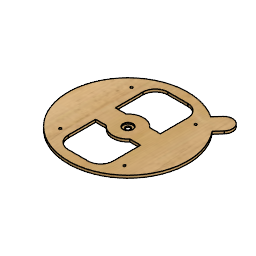
LB3 - Bucket Adapter (Autodesk Fusion 360 design; units mm, degrees)
Autodesk Fusion 360 part; units mm, degrees
sketch "Sketch1" plane through (0, 0, 0) normal (0, 0, 1) x (1, 0, 0)
  circle A0 centre (-64.5, 71.5) radius 2.25
  circle A1 centre (64.5, 71.5) radius 2.25
  circle A2 centre (-64.5, -71.5) radius 2.25
  circle A3 centre (64.5, -71.5) radius 2.25
  line L0 (20, 100) -> (-20, 100)
  line L1 (-20, -100) -> (20, -100)
  arc A4 (-20, 100) -> (-45, 75) centre (-20, 75) ccw
  arc A5 (45, 75) -> (20, 100) centre (20, 75) ccw
  arc A6 (20, -100) -> (45, -75) centre (20, -75) ccw
  arc A7 (-45, -75) -> (-20, -100) centre (-20, -75) ccw
  line L2 (45, 20) -> (-45, -20) construction
  circle A8 centre (0, 0) radius 5
  line L3 (64.5, 71.5) -> (-64.5, 71.5) construction
  line L4 (-64.5, 71.5) -> (-64.5, -71.5) construction
  line L5 (-64.5, -71.5) -> (64.5, -71.5) construction
  line L6 (64.5, -71.5) -> (64.5, 71.5) construction
  line L7 (64.5, 71.5) -> (-64.5, -71.5) construction
  line L8 (-64.5, 71.5) -> (64.5, -71.5) construction
  line L9 (45, 20) -> (23.6854, 20)
  line L10 (-23.6854, 20) -> (-45, 20)
  line L11 (-45, 75) -> (-45, 20)
  line L12 (-45, -20) -> (-45, -75)
  arc A9 (-23.6854, -20) -> (23.6854, -20) centre (0, 0) ccw
  arc A10 (23.6854, 20) -> (-23.6854, 20) centre (0, 0) ccw
  line L13 (45, -75) -> (45, -20)
  line L14 (45, 20) -> (45, 75)
  line L15 (-45, 20) -> (4.5691, -2.0307) construction
  line L16 (28.3282, -12.5903) -> (45, -20) construction
  line L17 (-45, -20) -> (-23.6854, -20)
  line L18 (23.6854, -20) -> (45, -20)
  line L19 (91.0962, 100.9826) -> (104.4615, 88.9257) construction
  line L20 (91.0962, 100.9826) -> (77.7308, 113.0394) construction
  line L21 (104.4615, 88.9257) -> (92.8349, 76.0373)
  line L22 (77.7308, 113.0394) -> (66.1042, 100.151)
  arc A11 (104.4615, 88.9257) -> (77.7308, 113.0394) centre (91.0962, 100.9826) ccw
  arc A12 (66.1042, 100.151) -> (92.8349, 76.0373) centre (0, 0) ccw
  dimension "d14" = 4.5
  dimension "d15" = 4.5
  dimension "d16" = 4.5
  dimension "d17" = 4.5
  dimension "d20" = 240
  dimension "d21" = 25
  dimension "d23" = 40
  dimension "d24" = 10
  dimension "d25" = 62
  dimension "d26" = 129
  dimension "d27" = 143
  dimension "d29" = 36
  dimension "d33" = 45
  dimension "d34" = 100
  dimension "d35" = 100
  dimension "d36" = 149.4615
  dimension "d37" = 132.054
  dimension "d38" = 213.0394
  dimension "d39" = 18.2443
  dimension "d40" = 18
  constraint horizontal L0
  constraint perpendicular L0 L11
  constraint parallel L0 L1
  constraint parallel L11 L13
  constraint tangent L0 A4
  constraint tangent A4 L11
  constraint tangent A5 L13
  constraint tangent L0 A5
  constraint equal A4 A5
  constraint tangent L1 A6
  constraint tangent A6 L13
  constraint equal A4 A6
  constraint tangent A7 L11
  constraint tangent L1 A7
  constraint equal A4 A7
  constraint horizontal L9
  constraint parallel L9 L17
  constraint coincident L2 A8.centre
  constraint coincident A8.centre L15
  constraint coincident A8.centre A9.centre
  constraint concentric A8 A12
  constraint horizontal L3
  constraint perpendicular L3 L4
  constraint parallel L3 L5
  constraint parallel L4 L6
  constraint coincident L7 A8.centre
  constraint coincident L8 A8.centre
  constraint collinear L9 L10
  constraint coincident L10.start A9
  constraint coincident L9.end A9
  constraint collinear L11 L12
  constraint coincident L16.start L15
  constraint concentric A9 A10
  constraint collinear L13 L14
  constraint coincident A8 L15.end
  constraint collinear L15 L16
  constraint coincident A9.end L17
  constraint collinear L17 L18
  constraint coincident L19.start L20.start
  constraint tangent L21 A11
  constraint tangent L22 A11
  constraint concentric A8 A9
  constraint coincident A2.centre L4.end
  constraint coincident A1.centre L3.start
  constraint coincident A3.centre L5.end
  constraint coincident A0.centre L3.end
  measures "d14" diameter of A0
  measures "d15" diameter of A1
  measures "d16" diameter of A2
  measures "d17" diameter of A3
  measures "d20" diameter of A12
  measures "d21" radius of A4
  measures "d23" distance of L10.end L2.end
  measures "d24" diameter of A8
  measures "d25" diameter of A9
  measures "d26" distance of A2.centre A3.centre
  measures "d27" distance of A0.centre A2.centre
  measures "d29" diameter of A11
  measures "d33" distance of A8.centre L11
  measures "d34" distance of A8.centre L1
  measures "d35" distance of A8.centre L0
  measures "d36" distance of L11 L19.end
  measures "d37" angle of L3 L21
  measures "d38" distance of L1 L20.end
  measures "d39" distance of L13.end L16.start
  measures "d40" distance of L7 L21
extrude "Extrude1" add sketch "Sketch1" along normal blind 5.2
sketch "Sketch4" plane through (0, 0, 5.2) normal (0, 0, 1) x (-1, 0, 0)
  circle A0 centre (-64.5, 71.5) radius 2.25
  circle A1 centre (64.5, 71.5) radius 2.25
  line L0 (-45, -20) -> (-23.6854, -20)
  arc A2 (-23.6854, -20) -> (23.6854, -20) centre (0, 0) ccw
  line L1 (23.6854, -20) -> (45, -20)
  line L2 (45, -20) -> (45, -75)
  arc A3 (20, -100) -> (45, -75) centre (20, -75) ccw
  line L3 (20, -100) -> (-20, -100)
  arc A4 (-45, -75) -> (-20, -100) centre (-20, -75) ccw
  line L4 (-45, -75) -> (-45, -20)
  circle A5 centre (64.5, -71.5) radius 2.25
  circle A6 centre (0, 0) radius 5
  line L5 (45, 75) -> (45, 20)
  line L6 (45, 20) -> (23.6854, 20)
  arc A7 (23.6854, 20) -> (-23.6854, 20) centre (0, 0) ccw
  line L7 (-23.6854, 20) -> (-45, 20)
  line L8 (-45, 20) -> (-45, 75)
  arc A8 (-20, 100) -> (-45, 75) centre (-20, 75) ccw
  line L9 (-20, 100) -> (20, 100)
  arc A9 (45, 75) -> (20, 100) centre (20, 75) ccw
  circle A10 centre (-64.5, -71.5) radius 2.25
  arc A11 (-104.4615, -88.9257) -> (-77.7308, -113.0394) centre (-91.0962, -100.9826) ccw
  line L10 (-77.7308, -113.0394) -> (-66.1042, -100.151)
  arc A12 (-66.1042, -100.151) -> (-92.8349, -76.0373) centre (0, 0) ccw
  line L11 (-92.8349, -76.0373) -> (-104.4615, -88.9257)
  circle A13 centre (0, 0) radius 10
  dimension "d30" = 20
  constraint concentric A2 A13
  measures "d30" diameter of A13
extrude "Extrude3" cut sketch "Sketch4" against normal blind 2.6 contours A13
equation "d31 = ( -5.2 / 2 ) * 1 mm"
